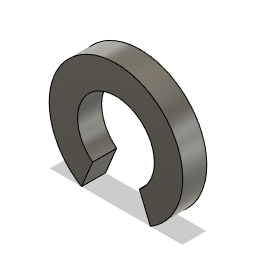
C Clip v1 (Autodesk Fusion 360 design; units mm, degrees)
Autodesk Fusion 360 part; units mm, degrees
sketch "Sketch1" plane through (0, 0, 0) normal (0, 0, 1) x (1, 0, 0)
  line L0 (-1.75, -2.281) -> (-2.5794, -4.2833)
  line L1 (1.75, -2.281) -> (2.5794, -4.2833)
  line L2 (0, 0) -> (0, -5) construction
  arc A0 (2.5794, -4.2833) -> (-2.5794, -4.2833) centre (0, 0) ccw
  arc A1 (1.75, -2.281) -> (-1.75, -2.281) centre (0, 0) ccw
  dimension "d7" = 5.75
  dimension "d8" = 10
  dimension "d9" = 45
  dimension "d10" = 3.5
  constraint coincident L2.start A0.centre
  constraint concentric A0 A1
  constraint vertical L2
  constraint symmetric L0 L1 L2
  measures "d7" diameter of A1
  measures "d8" diameter of A0
  measures "d9" angle of L0 L1
  measures "d10" distance of L1.start L0.start
extrude "Extrude1" add sketch "Sketch1" along normal blind 1.8
